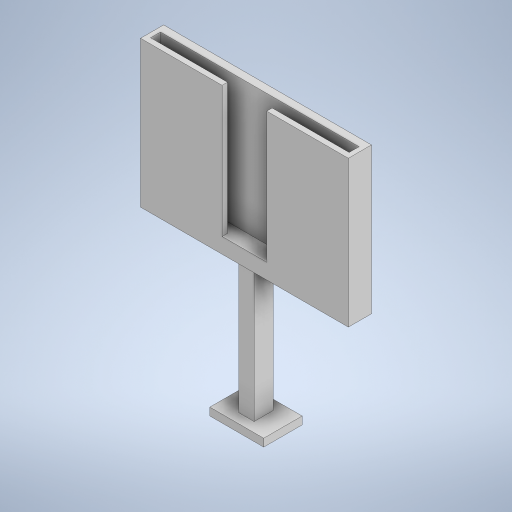
# Autodesk Inventor part: Inner Circle Landing Legs
Saved by Autodesk Inventor 2023 (Build 270158000, 158)
## iProperties
Created: 2022-12-04
Part Number: Inner Circle Landing Legs
Material: Generic
Document SubType Name: Modeling
Designer: cheng
Density: 1 g/cm^3
Appearance: Default
Author: cheng
Autodesk Inventor part; units mm, degrees
ref_plane "YZ Plane" through (0, 0, 0) normal (1, 0, 0) x (0, 1, 0)
ref_plane "XZ Plane" through (0, 0, 0) normal (0, 1, 0) x (-1, 0, 0)
ref_plane "XY Plane" through (0, 0, 0) normal (0, 0, 1) x (1, 0, 0)
sketch "Sketch1" plane through (0, 0, 0) normal (0, 1, 0) x (-1, 0, 0)
  line L0 (35, -25) -> (-35, -25)
  line L1 (-35, -25) -> (-35, 25)
  line L2 (-35, 25) -> (35, 25)
  line L3 (35, 25) -> (35, -25)
  line L4 (35, -25) -> (-35, 25) construction
  line L5 (-35, -25) -> (35, 25) construction
  point P0 (0, 0)
  dimension "d0" = 50
  dimension "d1" = 70
  constraints: 12 end point, 2 midpoint, 2 parallel, 1 horizontal, 1 perpendicular
  measures "d0" distance of L2.end L0.start
  measures "d1" distance of L0.start L0.end
extrude "Extrusion1" add sketch "Sketch1" along normal blind 10
sketch "Sketch2" plane through (0, 10, 0) normal (0, 1, 0) x (1, 0, 0)
  line L0 (10, -12.5) -> (-10, -12.5)
  line L1 (-10, -12.5) -> (-10, 12.5)
  line L2 (-10, 12.5) -> (10, 12.5)
  line L3 (10, 12.5) -> (10, -12.5)
  line L4 (10, -12.5) -> (-10, 12.5) construction
  line L5 (-10, -12.5) -> (10, 12.5) construction
  point P0 (0, 0)
  dimension "d4" = 20
  dimension "d5" = 25
  constraints: 12 end point, 2 midpoint, 2 parallel, 1 horizontal, 1 perpendicular
  measures "d4" distance of L1.end L2.end
  measures "d5" distance of L2.end L0.start
extrude "Extrusion2" add sketch "Sketch2" along normal blind 170
sketch "Sketch3" plane through (0, 180, 0) normal (0, 1, 0) x (1, 0, 0)
  line L0 (135, -15) -> (-135, -15)
  line L1 (-135, -15) -> (-135, 15)
  line L2 (-135, 15) -> (135, 15)
  line L3 (135, 15) -> (135, -15)
  line L4 (135, -15) -> (-135, 15) construction
  line L5 (-135, -15) -> (135, 15) construction
  point P0 (0, 0)
  dimension "d8" = 30
  dimension "d9" = 270
  constraints: 12 end point, 2 midpoint, 2 parallel, 1 horizontal, 1 perpendicular
  measures "d8" distance of L2.end L0.start
  measures "d9" distance between parallel lines of L1 L3
extrude "Extrusion3" add sketch "Sketch3" along normal blind 20
sketch "Sketch4" plane through (0, 200, 0) normal (0, 1, 0) x (1, 0, 0)
  line L0 (135, 15) -> (-135, 15) projected
  line L1 (-135, 15) -> (-135, -15) projected
  line L2 (-135, -15) -> (135, -15) projected
  line L3 (135, -15) -> (135, 15) projected
  line L4 (135, -15) -> (135, 15) projected
  line L5 (-135, 15) -> (-135, -15) projected
  line L6 (135, 15) -> (-135, 15)
  line L7 (-135, 15) -> (-135, 5)
  line L8 (-135, 5) -> (135, 5)
  line L9 (135, 5) -> (135, 15)
  line L10 (-135, -15) -> (135, -15) projected
  line L11 (-129, -15) -> (-135, -15)
  line L12 (-135, -15) -> (-135, 5)
  line L13 (-135, 5) -> (-129, 5)
  line L14 (-129, 5) -> (-129, -15)
  line L15 (129, -15) -> (135, -15)
  line L16 (135, -15) -> (135, 5)
  line L17 (135, 5) -> (129, 5)
  line L18 (129, 5) -> (129, -15)
  line L19 (129, -8) -> (29, -8)
  line L20 (29, -8) -> (29, -15)
  line L21 (29, -15) -> (129, -15)
  line L22 (129, -15) -> (129, -8)
  line L23 (-29, -15) -> (-129, -15)
  line L24 (-129, -15) -> (-129, -8)
  line L25 (-129, -8) -> (-29, -8)
  line L26 (-29, -8) -> (-29, -15)
  point P0 (0, 0)
  point P1 (-129, 5)
  dimension "d12" = 10
  dimension "d13" = 6
  dimension "d14" = 7
  dimension "d15" = 6
  dimension "d16" = 100
  dimension "d17" = 100
  dimension "d18" = 7
  constraints: 40 end point, 10 parallel, 8 point on line, 5 horizontal, 5 perpendicular
  measures "d12" distance between parallel lines of L0 L8
  measures "d13" distance between parallel lines of L1 L14
  measures "d14" distance between parallel lines of L25 L2
  measures "d15" distance between parallel lines of L3 L18
  measures "d16" distance of L19.start L19.end
  measures "d17" distance between parallel lines of L24 L26
  measures "d18" distance between parallel lines of L2 L19
extrude "Extrusion4" add sketch "Sketch4" along normal blind 170 contours L3 L8 L1 L0 | L3 L2 L18 L8 | L8 L14 L2 L1 | L2 L20 L19 L18 | L14 L25 L26 L2
body "Solid1"
